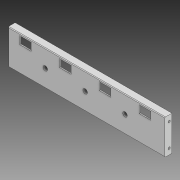
# Autodesk Inventor part: SensorHolder
Saved by Autodesk Inventor 2020 (Build 240168000, 168)
## iProperties
Created: 2020-12-18
Part Number: SensorHolder
Material: Generic
Document SubType Name: Modeling
Designer: DDeGo
Density: 1 g/cm^3
Appearance: Default
Author: DDeGo
Autodesk Inventor part; units mm, degrees
ref_plane "YZ Plane" through (0, 0, 0) normal (1, 0, 0) x (0, 1, 0)
ref_plane "XZ Plane" through (0, 0, 0) normal (0, 1, 0) x (-1, 0, 0)
ref_plane "XY Plane" through (0, 0, 0) normal (0, 0, 1) x (1, 0, 0)
sketch "Sketch1" plane through (0, 0, 0) normal (0, 0, 1) x (1, 0, 0)
  line L0 (-122, 13.5) -> (122, 13.5)
  line L1 (122, 13.5) -> (122, -13.5)
  line L2 (122, -13.5) -> (-122, -13.5)
  line L3 (-122, -13.5) -> (-122, 13.5)
  line L4 (-122, 13.5) -> (122, -13.5) construction
  line L5 (122, 13.5) -> (-122, -13.5) construction
  line L6 (-120.5, -12) -> (-96.5, -12)
  line L7 (-96.5, -12) -> (-96.5, 12)
  line L8 (-96.5, 12) -> (-120.5, 12)
  line L9 (-120.5, 12) -> (-120.5, -12)
  line L10 (-120.5, -12) -> (-96.5, 12) construction
  line L11 (-96.5, -12) -> (-120.5, 12) construction
  line L12 (-122, 0) -> (-108.5, 0) construction
  line L13 (-89.5, -12) -> (-65.5, -12)
  line L14 (-65.5, -12) -> (-65.5, 12)
  line L15 (-65.5, 12) -> (-89.5, 12)
  line L16 (-89.5, 12) -> (-89.5, -12)
  line L17 (-89.5, -12) -> (-65.5, 12) construction
  line L18 (-65.5, -12) -> (-89.5, 12) construction
  line L19 (-58.5, -12) -> (-34.5, -12)
  line L20 (-34.5, -12) -> (-34.5, 12)
  line L21 (-34.5, 12) -> (-58.5, 12)
  line L22 (-58.5, 12) -> (-58.5, -12)
  line L23 (-58.5, -12) -> (-34.5, 12) construction
  line L24 (-34.5, -12) -> (-58.5, 12) construction
  line L25 (-27.5, -12) -> (-3.5, -12)
  line L26 (-3.5, -12) -> (-3.5, 12)
  line L27 (-3.5, 12) -> (-27.5, 12)
  line L28 (-27.5, 12) -> (-27.5, -12)
  line L29 (-27.5, -12) -> (-3.5, 12) construction
  line L30 (-3.5, -12) -> (-27.5, 12) construction
  line L31 (3.5, -12) -> (27.5, -12)
  line L32 (27.5, -12) -> (27.5, 12)
  line L33 (27.5, 12) -> (3.5, 12)
  line L34 (3.5, 12) -> (3.5, -12)
  line L35 (3.5, -12) -> (27.5, 12) construction
  line L36 (27.5, -12) -> (3.5, 12) construction
  line L37 (34.5, -12) -> (58.5, -12)
  line L38 (58.5, -12) -> (58.5, 12)
  line L39 (58.5, 12) -> (34.5, 12)
  line L40 (34.5, 12) -> (34.5, -12)
  line L41 (34.5, -12) -> (58.5, 12) construction
  line L42 (58.5, -12) -> (34.5, 12) construction
  line L43 (65.5, -12) -> (89.5, -12)
  line L44 (89.5, -12) -> (89.5, 12)
  line L45 (89.5, 12) -> (65.5, 12)
  line L46 (65.5, 12) -> (65.5, -12)
  line L47 (65.5, -12) -> (89.5, 12) construction
  line L48 (89.5, -12) -> (65.5, 12) construction
  line L49 (96.5, -12) -> (120.5, -12)
  line L50 (120.5, -12) -> (120.5, 12)
  line L51 (120.5, 12) -> (96.5, 12)
  line L52 (96.5, 12) -> (96.5, -12)
  line L53 (96.5, -12) -> (120.5, 12) construction
  line L54 (120.5, -12) -> (96.5, 12) construction
  point P0 (0, 0)
  point P1 (-77.5, 0)
  point P2 (-46.5, 0)
  point P3 (-15.5, 0)
  point P4 (15.5, 0)
  point P5 (46.5, 0)
  point P6 (77.5, 0)
  point P7 (108.5, 0)
  dimension "d2" = 24
  dimension "d3" = 24
  dimension "d6" = 31
  dimension "d11" = 7
  dimension "d12" = 1.5
  dimension "d13" = 1.5
  dimension "d14" = 1.5
  constraints: 110 end point, 19 midpoint, 4 horizontal, 4 parallel, 2 perpendicular, 77 other
  measures "d2" distance of L7.end L8.end
  measures "d3" distance of L6.end L7.end
  measures "d6" distance of L6.start L13.start
  measures "d11" distance between parallel lines of L16 L7
  measures "d12" distance between parallel lines of L3 L9
  measures "d13" distance between parallel lines of L0 L8
  measures "d14" distance between parallel lines of L1 L50
extrude "Extrusion1" add sketch "Sketch1" along normal blind 4.5
sketch "Sketch2" plane through (0, 0, 4.5) normal (0, 0, 1) x (1, 0, 0)
  line L0 (-120.5, 12) -> (-96.5, 12) construction
  line L1 (-113, 6) -> (-104, 6)
  line L2 (-104, 6) -> (-104, 12)
  line L3 (-104, 12) -> (-113, 12)
  line L4 (-113, 12) -> (-113, 6)
  line L5 (-113, 6) -> (-104, 12) construction
  line L6 (-104, 6) -> (-113, 12) construction
  line L7 (-108.5, 12) -> (-108.5, 9) construction
  line L8 (122, 13.5) -> (-122, 13.5) projected
  line L9 (-122, -13.5) -> (122, -13.5) projected
  line L10 (-122, 13.5) -> (122, 13.5)
  line L11 (122, 13.5) -> (122, -13.5)
  line L12 (122, -13.5) -> (-122, -13.5)
  line L13 (-122, -13.5) -> (-122, 13.5)
  line L14 (-82, 6) -> (-73, 6)
  line L15 (-73, 6) -> (-73, 12)
  line L16 (-73, 12) -> (-82, 12)
  line L17 (-82, 12) -> (-82, 6)
  line L18 (-82, 6) -> (-73, 12) construction
  line L19 (-73, 6) -> (-82, 12) construction
  line L20 (-77.5, 12) -> (-77.5, 9) construction
  line L21 (-51, 6) -> (-42, 6)
  line L22 (-42, 6) -> (-42, 12)
  line L23 (-42, 12) -> (-51, 12)
  line L24 (-51, 12) -> (-51, 6)
  line L25 (-51, 6) -> (-42, 12) construction
  line L26 (-42, 6) -> (-51, 12) construction
  line L27 (-46.5, 12) -> (-46.5, 9) construction
  line L28 (-20, 6) -> (-11, 6)
  line L29 (-11, 6) -> (-11, 12)
  line L30 (-11, 12) -> (-20, 12)
  line L31 (-20, 12) -> (-20, 6)
  line L32 (-20, 6) -> (-11, 12) construction
  line L33 (-11, 6) -> (-20, 12) construction
  line L34 (-15.5, 12) -> (-15.5, 9) construction
  line L35 (11, 6) -> (20, 6)
  line L36 (20, 6) -> (20, 12)
  line L37 (20, 12) -> (11, 12)
  line L38 (11, 12) -> (11, 6)
  line L39 (11, 6) -> (20, 12) construction
  line L40 (20, 6) -> (11, 12) construction
  line L41 (15.5, 12) -> (15.5, 9) construction
  line L42 (42, 6) -> (51, 6)
  line L43 (51, 6) -> (51, 12)
  line L44 (51, 12) -> (42, 12)
  line L45 (42, 12) -> (42, 6)
  line L46 (42, 6) -> (51, 12) construction
  line L47 (51, 6) -> (42, 12) construction
  line L48 (46.5, 12) -> (46.5, 9) construction
  line L49 (73, 6) -> (82, 6)
  line L50 (82, 6) -> (82, 12)
  line L51 (82, 12) -> (73, 12)
  line L52 (73, 12) -> (73, 6)
  line L53 (73, 6) -> (82, 12) construction
  line L54 (82, 6) -> (73, 12) construction
  line L55 (77.5, 12) -> (77.5, 9) construction
  line L56 (104, 6) -> (113, 6)
  line L57 (113, 6) -> (113, 12)
  line L58 (113, 12) -> (104, 12)
  line L59 (104, 12) -> (104, 6)
  line L60 (104, 6) -> (113, 12) construction
  line L61 (113, 6) -> (104, 12) construction
  line L62 (108.5, 12) -> (108.5, 9) construction
  line L63 (-89.5, 12) -> (-65.5, 12) construction
  line L64 (-89.5, 12) -> (-65.5, 12) construction
  point P0 (0, 0)
  dimension "d17" = 6
  dimension "d18" = 9
  dimension "d21" = 31
  constraints: 120 end point, 19 midpoint, 4 parallel, 3 horizontal, 2 perpendicular, 1 coincident, 1 point on line, 1 vertical, 91 other
  measures "d17" distance of L1.end L2.end
  measures "d18" distance of L1.start L1.end
  measures "d21" distance of L1.start L14.start
extrude "Extrusion2" add sketch "Sketch2" along normal blind 1
sketch "Sketch3" plane through (0, 0, 0) normal (0, 0, -1) x (-1, 0, 0)
  line L0 (-96.5, -12) -> (-96.5, 12) projected
  line L1 (-96.5, 0) -> (-89.5, 0) construction
  line L2 (-89.5, 12) -> (-89.5, -12) projected
  circle A0 centre (-93, 0) radius 1.75
  line L3 (-65.5, -12) -> (-65.5, 12) projected
  line L4 (-65.5, 0) -> (-58.5, 0) construction
  line L5 (-58.5, 12) -> (-58.5, -12) projected
  circle A1 centre (-62, 0) radius 1.75
  circle A2 centre (-31, 0) radius 1.75
  circle A3 centre (0, 0) radius 1.75
  circle A4 centre (31, 0) radius 1.75
  circle A5 centre (62, 0) radius 1.75
  circle A6 centre (93, 0) radius 1.75
  point P0 (0, 0)
  dimension "d28" = 3.5
  dimension "d31" = 31
  constraints: 7 centre point, 6 midpoint, 4 end point, 1 horizontal, 12 other
  measures "d28" diameter of A0
  measures "d31" distance of A0.centre A1.centre
extrude "Extrusion3" cut sketch "Sketch3" against normal through all contours A0 | A1 | A2 | A4 | A5 | A6
sketch "Sketch4" plane through (-122, -13.5, 0) normal (0, -1, 0) x (1, 0, 0)
  line L0 (242.5, 0) -> (218.5, 0) projected
  line L1 (211.5, 0) -> (187.5, 0) projected
  line L2 (231.5, 1) -> (229.5, 1)
  line L3 (229.5, 1) -> (229.5, -1)
  line L4 (229.5, -1) -> (231.5, -1)
  line L5 (231.5, -1) -> (231.5, 1)
  line L6 (231.5, 1) -> (229.5, -1) construction
  line L7 (229.5, 1) -> (231.5, -1) construction
  line L8 (200.5, 1) -> (198.5, 1)
  line L9 (198.5, 1) -> (198.5, -1)
  line L10 (198.5, -1) -> (200.5, -1)
  line L11 (200.5, -1) -> (200.5, 1)
  line L12 (200.5, 1) -> (198.5, -1) construction
  line L13 (198.5, 1) -> (200.5, -1) construction
  line L14 (169.5, 1) -> (167.5, 1)
  line L15 (167.5, 1) -> (167.5, -1)
  line L16 (167.5, -1) -> (169.5, -1)
  line L17 (169.5, -1) -> (169.5, 1)
  line L18 (169.5, 1) -> (167.5, -1) construction
  line L19 (167.5, 1) -> (169.5, -1) construction
  line L20 (138.5, 1) -> (136.5, 1)
  line L21 (136.5, 1) -> (136.5, -1)
  line L22 (136.5, -1) -> (138.5, -1)
  line L23 (138.5, -1) -> (138.5, 1)
  line L24 (138.5, 1) -> (136.5, -1) construction
  line L25 (136.5, 1) -> (138.5, -1) construction
  line L26 (107.5, 1) -> (105.5, 1)
  line L27 (105.5, 1) -> (105.5, -1)
  line L28 (105.5, -1) -> (107.5, -1)
  line L29 (107.5, -1) -> (107.5, 1)
  line L30 (107.5, 1) -> (105.5, -1) construction
  line L31 (105.5, 1) -> (107.5, -1) construction
  line L32 (76.5, 1) -> (74.5, 1)
  line L33 (74.5, 1) -> (74.5, -1)
  line L34 (74.5, -1) -> (76.5, -1)
  line L35 (76.5, -1) -> (76.5, 1)
  line L36 (76.5, 1) -> (74.5, -1) construction
  line L37 (74.5, 1) -> (76.5, -1) construction
  line L38 (45.5, 1) -> (43.5, 1)
  line L39 (43.5, 1) -> (43.5, -1)
  line L40 (43.5, -1) -> (45.5, -1)
  line L41 (45.5, -1) -> (45.5, 1)
  line L42 (45.5, 1) -> (43.5, -1) construction
  line L43 (43.5, 1) -> (45.5, -1) construction
  line L44 (14.5, 1) -> (12.5, 1)
  line L45 (12.5, 1) -> (12.5, -1)
  line L46 (12.5, -1) -> (14.5, -1)
  line L47 (14.5, -1) -> (14.5, 1)
  line L48 (14.5, 1) -> (12.5, -1) construction
  line L49 (12.5, 1) -> (14.5, -1) construction
  point P0 (122, 0)
  point P1 (230.5, 0)
  point P2 (199.5, 0)
  point P3 (168.5, 0)
  point P4 (137.5, 0)
  point P5 (106.5, 0)
  point P6 (75.5, 0)
  point P7 (44.5, 0)
  point P8 (13.5, 0)
  dimension "d40" = 31
  dimension "d45" = 1
  dimension "d46" = 2
  constraints: 96 end point, 18 midpoint, 2 horizontal, 2 parallel, 1 perpendicular, 77 other
  measures "d40" distance of L2.start L8.start
  measures "d45" distance between parallel lines of L2 L0
  measures "d46" distance of L2.start L2.end
extrude "Extrusion4" cut sketch "Sketch4" against normal blind 4.5
sketch "Sketch5" plane through (-3.5, -12, 0) normal (-1, 0, 0) x (0, 0, 1)
  line L0 (0, 0) -> (4.5, 0) projected
  line L1 (2.25, 0) -> (2.25, 24) construction
  line L2 (0, 24) -> (4.5, 24) projected
  circle A0 centre (2.25, 3) radius 0.85
  circle A1 centre (2.25, 21) radius 0.85
  point P0 (0, 12)
  dimension "d49" = 1.7
  dimension "d50" = 3
  dimension "d51" = 3
  constraints: 2 centre point, 2 end point, 2 midpoint, 2 point on line, 1 equal radius
  measures "d49" diameter of A0
  measures "d50" distance from line of L2 A1.centre
  measures "d51" distance from line of A0.centre L0
extrude "Extrusion5" cut sketch "Sketch5" against normal up to surface (7 mm away)
chamfer "Chamfer1" distance 0.5 angle 45 4 edges at (0, -13.5, 5.5) (122, 0, 5.5) (0, 13.5, 5.5) (-122, 0, 5.5)
sketch "Sketch7" plane through (0, 0, 0) normal (0, 0, -1) x (-1, 0, 0)
  line L0 (-167.9022, 73.2731) -> (0, 73.2731)
  line L1 (0, 73.2731) -> (0, -62.2269)
  line L2 (0, -62.2269) -> (-167.9022, -62.2269)
  line L3 (-167.9022, -62.2269) -> (-167.9022, 73.2731)
  line L4 (0, 73.2731) -> (150.1362, 73.2731)
  line L5 (150.1362, 73.2731) -> (150.1362, -62.2269)
  line L6 (150.1362, -62.2269) -> (0, -62.2269)
  line L7 (0, -62.2269) -> (0, 73.2731)
  point P0 (0, 0)
  constraints: 16 end point, 4 parallel, 2 horizontal, 2 perpendicular, 1 point on line
extrude "Extrusion7" cut sketch "Sketch7" against normal through all contours L0 L1 L2 L3
body "Solid1"
